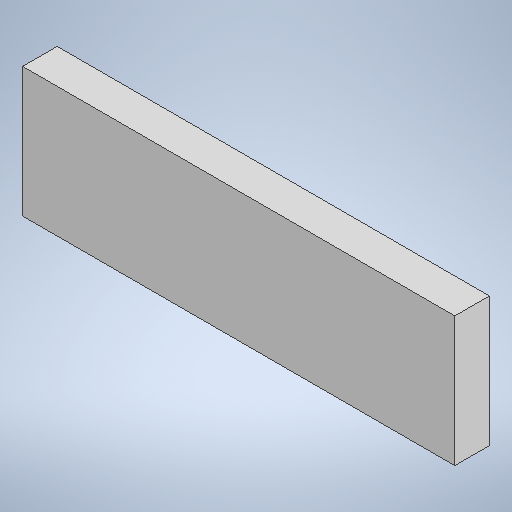
# Autodesk Inventor part: Peça12
Saved by Autodesk Inventor 2025.2 (Build 292293000, 293)
## iProperties
Created: 2025-05-31
Part Number: Peça12
Material: Genérico
Document SubType Name: Modeling
Designer: Gustavo Sousa
Density: 1 g/cm^3
Appearance: Padrão
Author: Gustavo Sousa
Autodesk Inventor part; units mm, degrees
ref_plane "YZ Plane" through (0, 0, 0) normal (1, 0, 0) x (0, 1, 0)
ref_plane "XZ Plane" through (0, 0, 0) normal (0, 1, 0) x (-1, 0, 0)
ref_plane "XY Plane" through (0, 0, 0) normal (0, 0, 1) x (1, 0, 0)
sketch "Esboço1" plane through (0, 0, 0) normal (0, 0, 1) x (1, 0, 0)
  line L0 (-25, -7.5) -> (25, -7.5)
  line L1 (25, -7.5) -> (25, 7.5)
  line L2 (25, 7.5) -> (-25, 7.5)
  line L3 (-25, 7.5) -> (-25, -7.5)
  line L4 (-25, -7.5) -> (25, 7.5) construction
  line L5 (25, -7.5) -> (-25, 7.5) construction
  point P0 (0, 0)
  dimension "d0" = 50
  dimension "d1" = 15
  constraints: 12 end point, 2 midpoint, 2 parallel, 1 horizontal, 1 perpendicular
  measures "d0" distance of L2.end L1.end
  measures "d1" distance of L0.end L1.end
extrude "Extrusão1" add sketch "Esboço1" along normal mid plane 4
